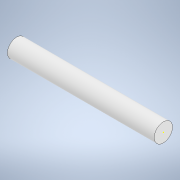
# Autodesk Inventor part: rod
Saved by Autodesk Inventor 2022 (Build 260153000, 153)
## iProperties
Created: 2023-06-18
Part Number: rod
Material: PVC-Piping
Document SubType Name: Modeling
Designer: Preeti Anand
Density: 1.4 g/cm^3
Appearance: Smooth - White
Author: Preeti Anand
Autodesk Inventor part; units mm, degrees
ref_plane "YZ Plane" through (0, 0, 0) normal (1, 0, 0) x (0, 1, 0)
ref_plane "XZ Plane" through (0, 0, 0) normal (0, 1, 0) x (-1, 0, 0)
ref_plane "XY Plane" through (0, 0, 0) normal (0, 0, 1) x (1, 0, 0)
sketch "Sketch1" plane through (0, 0, 0) normal (0, 0, 1) x (1, 0, 0)
  line L0 (0, 0) -> (80, 0)
  line L1 (80, 0) -> (80, 5)
  line L2 (80, 5) -> (0, 5)
  line L3 (0, 5) -> (0, 0)
  line L4 (-58.7875, 0) -> (108.1668, 0)
  dimension "d0" = 80
  dimension "d1" = 5
  constraints: 10 end point, 3 perpendicular, 2 horizontal
  measures "d0" distance of L0.start L0.end
  measures "d1" distance of L0.end L1.end
revolve "Revolution1" add sketch "Sketch1" angle 360 about axis through (-58.7875, 0, 0) along (1, 0, 0)
sketch "Sketch2" plane through (80, 0, 0) normal (1, 0, 0) x (0, 0, -1)
  point P0 (0, 0)
body "Solid1"
